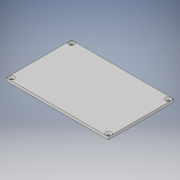
# Autodesk Inventor part: BoxLid
Saved by Autodesk Inventor 2019.4 (Build 234330000, 330)
## iProperties
Created: 2020-02-26
Part Number: BoxLid
Material: Generic
Document SubType Name: Modeling
Designer: ions
Density: 1 g/cm^3
Appearance: Default
Author: ions
Autodesk Inventor part; units mm, degrees
ref_plane "YZ Plane" through (0, 0, 0) normal (1, 0, 0) x (0, 1, 0)
ref_plane "XZ Plane" through (0, 0, 0) normal (0, 1, 0) x (-1, 0, 0)
ref_plane "XY Plane" through (0, 0, 0) normal (0, 0, 1) x (1, 0, 0)
sketch "Sketch1" plane through (0, 0, 0) normal (0, 1, 0) x (-1, 0, 0)
  line L0 (43.2913, 23.5582) -> (-30.2087, 23.5582)
  line L1 (-30.2087, 23.5582) -> (-30.2087, -23.4418)
  line L2 (-30.2087, -23.4418) -> (43.2913, -23.4418)
  line L3 (43.2913, -23.4418) -> (43.2913, 23.5582)
  point P0 (0, 0)
  dimension "d0" = 47
  dimension "d1" = 73.5
  constraints: 8 end point, 2 parallel, 1 horizontal, 1 perpendicular
  measures "d0" distance between parallel lines of L2 L0
  measures "d1" distance between parallel lines of L3 L1
extrude "Extrusion1" add sketch "Sketch1" along normal blind 2
sketch "Sketch2" plane through (0, 2, 0) normal (0, 1, 0) x (1, 0, 0)
  circle A0 centre (-41.2913, -21.5582) radius 0.8353
  line L0 (-43.2913, -23.5582) -> (30.2087, -23.5582) projected
  line L1 (-43.2913, 23.4418) -> (-43.2913, -23.5582) projected
  point P0 (0, 0)
  dimension "d4" = 2
  dimension "d5" = 2
  constraints: 1 centre point
  measures "d4" distance from line of L0 A0.centre
  measures "d5" distance from line of L1 A0.centre
hole "Hole1" at (-41.2913, 2, 21.5582) direction (0, -1, 0) diameter 1.694 depth 2 countersink diameter 4 countersink angle 90 thread size "2-56 UNC" class "2B" standard "ANSI Unified Screw Threads"
pattern_linear "Rectangular Pattern1" count 2 spacing 43 along (0, 0, -1) count 2 spacing 69.5 along (1, 0, 0) of "Hole1"
body "Solid1"
